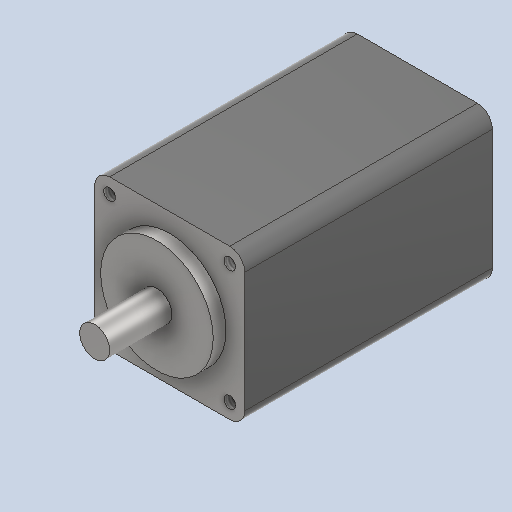
# Autodesk Inventor part: StepperMotor
Saved by Autodesk Inventor 2023 (Build 270158000, 158)
## iProperties
Created: 2022-12-26
Part Number: StepperMotor
Material: Generic
Document SubType Name: Modeling
Designer: karpova
Density: 1 g/cm^3
Appearance: Stainless - Brushed
Author: karpova
Autodesk Inventor part; units mm, degrees
ref_plane "YZ Plane" through (0, 0, 0) normal (1, 0, 0) x (0, 1, 0)
ref_plane "XZ Plane" through (0, 0, 0) normal (0, 1, 0) x (-1, 0, 0)
ref_plane "XY Plane" through (0, 0, 0) normal (0, 0, 1) x (1, 0, 0)
sketch "Sketch1" plane through (0, 0, 0) normal (0, 0, 1) x (1, 0, 0)
  line L0 (-8, 10) -> (8, 10)
  line L1 (10, 8) -> (10, -8)
  line L2 (8, -10) -> (-8, -10)
  line L3 (-10, -8) -> (-10, 8)
  line L4 (0, 0) -> (10, 0) construction
  line L5 (0, 0) -> (0, 10) construction
  arc A0 (-8, 10) -> (-10, 8) centre (-8, 8) ccw
  arc A1 (-10, -8) -> (-8, -10) centre (-8, -8) ccw
  arc A2 (8, -10) -> (10, -8) centre (8, -8) ccw
  arc A3 (10, 8) -> (8, 10) centre (8, 8) ccw
  point P0 (10, -10)
  point P1 (10, 10)
  dimension "d1" = 20
  dimension "d3" = 16
  constraints: 12 end point, 8 point on circle, 8 tangent, 4 centre point, 4 point on line, 3 equal radius, 2 horizontal, 2 midpoint, 2 parallel, 2 perpendicular, 1 vertical
  measures "d1" distance of point (10, 10) point (10, -10)
  measures "d3" distance of L1.start L1.end
extrude "Extrusion1" add sketch "Sketch1" along normal blind 33
sketch "Sketch2" plane through (0, 0, 33) normal (0, 0, 1) x (1, 0, 0)
  circle A0 centre (0, 0) radius 7.5
  dimension "d6" = 15
  constraints: 1 centre point, 1 coincident
  measures "d6" diameter of A0
extrude "Extrusion2" add sketch "Sketch2" along normal blind 1.7
sketch "Sketch3" plane through (0, 0, 34.7) normal (0, 0, 1) x (1, 0, 0)
  circle A0 centre (0, 0) radius 2
  dimension "d9" = 4
  constraints: 1 centre point, 1 coincident
  measures "d9" diameter of A0
extrude "Extrusion3" add sketch "Sketch3" along normal blind 10 from surface at -1.7
sketch "Sketch4" plane through (-8, -10, 0) normal (0, -1, 0) x (1, 0, 0)
  line L0 (16, 0) -> (0, 0) projected
  line L1 (2, 0) -> (14, 0)
  line L2 (14, 0) -> (14, 8)
  line L3 (8, 8) -> (2, 8)
  line L4 (2, 8) -> (2, 0)
  line L5 (8, 0) -> (8, 46.0613) construction
  line L6 (8, 8) -> (14, 8)
  dimension "d12" = 12
  dimension "d13" = 8
  constraints: 12 end point, 2 horizontal, 2 parallel, 2 point on line, 1 collinear, 1 perpendicular, 1 vertical
  measures "d12" distance between parallel lines of L2 L4
  measures "d13" distance between parallel lines of L0 L6
extrude "Extrusion4" add sketch "Sketch4" along normal blind 1.75
sketch "Sketch5" plane through (0, 0, 33) normal (0, 0, 1) x (1, 0, 0)
  line L0 (8, 10) -> (-8, 10) construction
  line L1 (6, -10) -> (8, -10) construction
  line L2 (-8, 10) -> (8, 10) construction
  line L3 (8, 10) -> (8, -10) construction
  line L4 (8, -10) -> (-8, -10) construction
  line L5 (-8, -10) -> (-8, 10) construction
  line L6 (10, -8) -> (10, 8) construction
  line L7 (-10, 8) -> (-10, -8) construction
  line L8 (10, 8) -> (-10, 8) construction
  line L9 (-10, 8) -> (-10, -8) construction
  line L10 (-10, -8) -> (10, -8) construction
  line L11 (10, -8) -> (10, 8) construction
  point P0 (0, 0)
  point P1 (-8, 8)
  point P2 (8, 8)
  point P3 (8, -8)
  point P4 (-8, -8)
  constraints: 16 end point, 8 point on line, 4 parallel, 2 horizontal, 2 perpendicular
hole "Hole1" at (-8, 8, 33) at (8, 8, 33) at (8, -8, 33) at (-8, -8, 33) direction (0, 0, -1) diameter 1.567 depth 8 thread size "M2x0.4" class "6H" standard "ANSI Metric M Profile"
sketch "Sketch6" plane through (0, 0, 0) normal (0, 0, -1) x (-1, 0, 0)
  line L0 (-4, -10.25) -> (4, -10.25)
  line L1 (4, -10.25) -> (4, -10.75)
  line L2 (-4, -10.75) -> (-4, -10.25)
  line L3 (0, 0) -> (0, -11.75) construction
  line L4 (-6, -11.75) -> (6, -11.75) construction
  line L5 (4, -10.75) -> (0, -10.75)
  line L6 (-4, -10.75) -> (0, -10.75)
  line L7 (8, -10) -> (-8, -10) projected
  dimension "d23" = 8
  dimension "d24" = 0.5
  dimension "d25" = 1
  constraints: 12 end point, 2 horizontal, 2 parallel, 1 collinear, 1 midpoint, 1 perpendicular, 1 point on line
  measures "d23" distance between parallel lines of L1 L2
  measures "d24" distance between parallel lines of L5 L0
  measures "d25" distance between parallel lines of L4 L5
extrude "Extrusion5" [suppressed]
equation "\"d13\" = extrusionHeight"
equation "\"d21\" = screwDepth"
equation "\"d23\" = ribbonWidth"
equation "\"d24\" = ribbonThickness"
equation "\"d25\" = ribbonEdgeOffset"
equation "\"extrusionHeight\" = 8"
equation "\"screwDepth\" = 8"
equation "\"ribbonWidth\" = 8"
equation "\"ribbonThickness\" = 0.5"
equation "\"ribbonEdgeOffset\" = 1"
body "Solid1"
